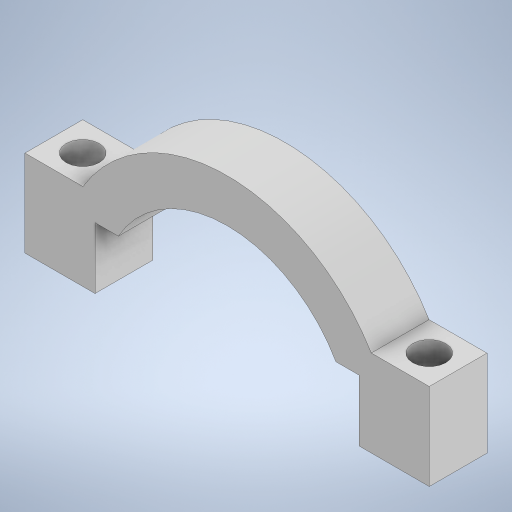
# Autodesk Inventor part: 가스벨브 상단 커버
Saved by Autodesk Inventor 2023.1 (Build 271208000, 208)
## iProperties
Created: 2022-08-17
Part Number: 가스벨브 상단 커버
Material: 일반
Document SubType Name: Modeling
Designer: fly01
Density: 1 g/cm^3
Appearance: 기본값
Author: fly01
Autodesk Inventor part; units mm, degrees
ref_plane "YZ Plane" through (0, 0, 0) normal (1, 0, 0) x (0, 1, 0)
ref_plane "XZ Plane" through (0, 0, 0) normal (0, 1, 0) x (-1, 0, 0)
ref_plane "XY Plane" through (0, 0, 0) normal (0, 0, 1) x (1, 0, 0)
sketch "스케치1" plane through (0, 0, 0) normal (0, 0, 1) x (1, 0, 0)
  line L0 (-14, 0) -> (14, 0)
  circle A0 centre (0, 0) radius 8.65
  line L1 (-9.15, 4.25) -> (9.15, 4.25)
  line L2 (9.15, 4.25) -> (9.15, -4.25)
  line L3 (9.15, -4.25) -> (-9.15, -4.25)
  line L4 (-9.15, -4.25) -> (-9.15, 4.25)
  line L5 (-9.15, 4.25) -> (9.15, -4.25) construction
  line L6 (9.15, 4.25) -> (-9.15, -4.25) construction
  line L7 (-14, 0) -> (-14, 6)
  line L8 (-14, 6) -> (-9.9861, 6)
  circle A1 centre (0, 0) radius 11.65
  line L9 (0, 0) -> (0, -1.5654)
  line L10 (14, 0) -> (14, 6)
  line L11 (14, 6) -> (9.9861, 6)
  point P0 (-9.15, 0)
  point P1 (-7.5339, 4.25)
  point P2 (7.5339, 4.25)
  point P3 (9.15, 0)
  dimension "d0" = 28
  dimension "d1" = 17.3
  dimension "d2" = 18.3
  dimension "d3" = 8.5
  dimension "d4" = 6
  dimension "d5" = 3
  constraints: 24 end point, 3 coincident, 3 midpoint, 2 horizontal, 2 parallel, 2 perpendicular, 2 symmetric about line, 2 vertical, 1 centre point, 3 other
  measures "d0" distance of L0.start L0.end
  measures "d1" diameter of A0
  measures "d2" distance of L2.end L3.end
  measures "d3" distance of L1.end L2.end
  measures "d4" distance of L0.start L7.end
extrude "돌출1" add sketch "스케치1" along normal blind 4 contours L2 L1 A0 L4 L0 A1 | A1 L11 L10 L0 | L0 L7 L8 A1
sketch "스케치2" plane through (-14, 6, 0) normal (0, 1, 0) x (1, 0, 0)
  line L0 (2, -2) -> (26, -2)
  line L1 (4.0139, 0) -> (0, 0) projected
  line L2 (4.0139, 0) -> (23.9861, 0) projected
  circle A0 centre (2, -2) radius 1.15
  circle A1 centre (26, -2) radius 1.15
  point P0 (14, 0)
  point P1 (14, -2)
  point P2 (14, 0)
  dimension "d8" = 2
  dimension "d9" = 24
  dimension "d10" = 2.3
  dimension "d11" = 2.3
  constraints: 2 centre point, 2 coincident, 2 end point, 2 midpoint, 1 horizontal, 1 vertical alignment
  measures "d8" distance between parallel lines of L1 L0
  measures "d9" distance of L0.start L0.end
  measures "d10" diameter of A0
  measures "d11" diameter of A1
extrude "돌출2" cut sketch "스케치2" against normal up to surface (6 mm away)
